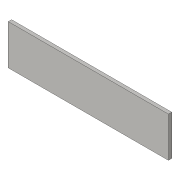
# Autodesk Inventor part: jh
Saved by Autodesk Inventor 2016 (Build 200138000, 138)
## iProperties
Created: 2018-01-26
Part Number: jh
Material: Generic
Document SubType Name: Modeling
Designer: lyonsp
Density: 1 g/cm^3
Appearance: Default
Author: lyonsp
Autodesk Inventor part; units mm, degrees
ref_plane "YZ Plane" through (0, 0, 0) normal (1, 0, 0) x (0, 1, 0)
ref_plane "XZ Plane" through (0, 0, 0) normal (0, 1, 0) x (-1, 0, 0)
ref_plane "XY Plane" through (0, 0, 0) normal (0, 0, 1) x (1, 0, 0)
sketch "Sketch1" plane through (0, 0, 0) normal (0, 0, 1) x (1, 0, 0)
  line L0 (-157.2381, 74.4721) -> (147.5619, 74.4721)
  line L1 (147.5619, 74.4721) -> (147.5619, -1.7279)
  line L2 (147.5619, -1.7279) -> (-157.2381, -1.7279)
  line L3 (-157.2381, -1.7279) -> (-157.2381, 74.4721)
  point P0 (0, 0)
  dimension "d0" = 304.8
  dimension "d1" = 76.2
  constraints: 8 end point, 2 parallel, 1 horizontal, 1 perpendicular
  measures "d0" distance of L0.start L0.end
  measures "d1" distance of L2.end L0.start
extrude "Extrusion1" add sketch "Sketch1" along normal blind 6.35
body "Solid1"
